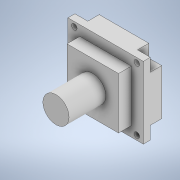
# Autodesk Inventor part: imx291CameraModule
Saved by Autodesk Inventor 2022.1 (Build 261234000, 234)
## iProperties
Created: 2021-07-20
Part Number: imx291CameraModule
Material: Generic
Document SubType Name: Modeling
Designer: robst
Density: 1 g/cm^3
Appearance: Default
Author: robst
Autodesk Inventor part; units mm, degrees
ref_plane "YZ Plane" through (0, 0, 0) normal (1, 0, 0) x (0, 1, 0)
ref_plane "XZ Plane" through (0, 0, 0) normal (0, 1, 0) x (-1, 0, 0)
ref_plane "XY Plane" through (0, 0, 0) normal (0, 0, 1) x (1, 0, 0)
sketch "Sketch1" plane through (0, 0, 0) normal (0, 0, 1) x (1, 0, 0)
  line L0 (-20.5, -19.5) -> (20.5, -19.5)
  line L1 (20.5, -19.5) -> (20.5, 19.5)
  line L2 (20.5, 19.5) -> (-20.5, 19.5)
  line L3 (-20.5, 19.5) -> (-20.5, -19.5)
  line L4 (-20.5, -19.5) -> (20.5, 19.5) construction
  line L5 (20.5, -19.5) -> (-20.5, 19.5) construction
  line L6 (-17, -17) -> (17, -17) construction
  line L7 (17, -17) -> (17, 17) construction
  line L8 (17, 17) -> (-17, 17) construction
  line L9 (-17, 17) -> (-17, -17) construction
  line L10 (-17, -17) -> (17, 17) construction
  line L11 (17, -17) -> (-17, 17) construction
  circle A0 centre (-17, 17) radius 1.5
  circle A1 centre (17, 17) radius 1.5
  circle A2 centre (17, -17) radius 1.5
  circle A3 centre (-17, -17) radius 1.5
  point P0 (0, 0)
  dimension "d0" = 41
  dimension "d1" = 39
  dimension "d2" = 34
  dimension "d3" = 34
  dimension "d4" = 3
  constraints: 24 end point, 5 coincident, 4 centre point, 4 midpoint, 4 parallel, 3 equal radius, 2 horizontal, 2 perpendicular
  measures "d0" distance of L1.end L2.end
  measures "d1" distance of L2.end L0.start
  measures "d2" distance of L7.end L8.end
  measures "d3" distance of L8.end L6.start
  measures "d4" diameter of A0
extrude "Extrusion1" add sketch "Sketch1" against normal blind 10
sketch "Sketch2" plane through (0, 0, 0) normal (0, 0, 1) x (1, 0, 0)
  line L0 (-14, -14) -> (14, -14)
  line L1 (14, -14) -> (14, 14)
  line L2 (14, 14) -> (-14, 14)
  line L3 (-14, 14) -> (-14, -14)
  line L4 (-14, -14) -> (14, 14) construction
  line L5 (14, -14) -> (-14, 14) construction
  point P0 (0, 0)
  dimension "d7" = 28
  dimension "d8" = 28
  constraints: 12 end point, 2 midpoint, 2 parallel, 1 horizontal, 1 perpendicular
  measures "d7" distance of L1.end L2.end
  measures "d8" distance of L2.end L0.start
extrude "Extrusion2" add sketch "Sketch2" along normal blind 7
sketch "Sketch3" plane through (0, 0, 7) normal (0, 0, 1) x (1, 0, 0)
  circle A0 centre (0, 0) radius 7.1
  dimension "d11" = 14.2
  constraints: 1 centre point, 1 coincident
  measures "d11" diameter of A0
extrude "Extrusion3" add sketch "Sketch3" along normal blind 20
sketch "Sketch4" plane through (0, 0, -10) normal (0, 0, -1) x (-1, 0, 0)
  line L0 (-20.5, 19.5) -> (-20.5, -19.5) projected
  line L1 (-20.5, 19.5) -> (-13.5, 19.5)
  line L2 (-13.5, 19.5) -> (-13.5, 12.5)
  line L3 (-13.5, 12.5) -> (-20.5, 12.5)
  line L4 (-20.5, 12.5) -> (-20.5, 19.5)
  line L5 (20.5, 19.5) -> (-20.5, 19.5) projected
  line L6 (20.5, 19.5) -> (13.5, 19.5)
  line L7 (13.5, 19.5) -> (13.5, 12.5)
  line L8 (13.5, 12.5) -> (20.5, 12.5)
  line L9 (20.5, 12.5) -> (20.5, 19.5)
  line L10 (20.5, 19.5) -> (20.5, -19.5) projected
  line L11 (20.5, -19.5) -> (13.5, -19.5)
  line L12 (13.5, -19.5) -> (13.5, -12.5)
  line L13 (13.5, -12.5) -> (20.5, -12.5)
  line L14 (20.5, -12.5) -> (20.5, -19.5)
  line L15 (-20.5, -19.5) -> (-13.5, -19.5)
  line L16 (-13.5, -19.5) -> (-13.5, -12.5)
  line L17 (-13.5, -12.5) -> (-20.5, -12.5)
  line L18 (-20.5, -12.5) -> (-20.5, -19.5)
  point P0 (0, 0)
  dimension "d14" = 7
  constraints: 32 end point, 8 parallel, 7 equal length, 4 horizontal, 4 perpendicular, 2 point on line
  measures "d14" distance of L0.start L1.end
extrude "Extrusion4" cut sketch "Sketch4" against normal blind 6.2
equation "\"d0\" = imx291ModuleWidth"
equation "\"d1\" = imx291ModuleLength"
equation "\"d2\" = imx291ModuleScrewWidthDistance"
equation "\"d3\" = imx291ModuleScrewLengthDistance"
equation "\"d4\" = screwDiameterHole"
equation "\"d5\" = imx291ModuleDepth"
equation "\"d7\" = lensBaseWidth"
equation "\"d8\" = lensBaseLength"
equation "\"d9\" = lensBaseDepth"
equation "\"d11\" = lensDiameter"
equation "\"d12\" = lensDepth"
equation "\"imx291ModuleWidth\" = 41"
equation "\"imx291ModuleLength\" = 39"
equation "\"imx291ModuleDepth\" = 10"
equation "\"imx291ModuleScrewWidthDistance\" = 34"
equation "\"imx291ModuleScrewLengthDistance\" = 34"
equation "\"screwDiameterHole\" = 3"
equation "\"lensBaseWidth\" = 28"
equation "\"lensBaseLength\" = 28"
equation "\"lensBaseDepth\" = 7"
equation "\"lensDiameter\" = 14.2"
equation "\"lensDepth\" = 20"
body "Solid1"
